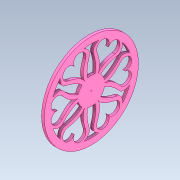
# Autodesk Inventor part: WheelFace
Saved by Autodesk Inventor 2021 (Build 250183000, 183)
## iProperties
Created: 2021-08-28
Part Number: WheelFace
Material: ABS Plastic
Document SubType Name: Modeling
Designer: digge
Density: 1.06 g/cm^3
Appearance: Pink
Author: digge
Autodesk Inventor part; units mm, degrees
ref_plane "YZ Plane" through (0, 0, 0) normal (1, 0, 0) x (0, 1, 0)
ref_plane "XZ Plane" through (0, 0, 0) normal (0, 1, 0) x (-1, 0, 0)
ref_plane "XY Plane" through (0, 0, 0) normal (0, 0, 1) x (1, 0, 0)
sketch "Sketch1" plane through (0, 0, 0) normal (1, 0, 0) x (0, 1, 0)
  circle A0 centre (168, 158) radius 175
  circle A1 centre (168, 158) radius 1.5
  point P0 (0, 0)
  dimension "d0" = 3
  dimension "d1" = 350
  constraints: 2 centre point, 1 coincident
  measures "d0" diameter of A1
  measures "d1" diameter of A0
extrude "Extrusion1" add sketch "Sketch1" along normal blind 10
sketch "Sketch2" plane through (10, 168, 158) normal (1, 0, 0) x (0, 0, -1)
  circle A0 centre (0, 0) radius 175 projected
  circle A1 centre (0, 0) radius 175 projected
  circle A2 centre (0, 0) radius 1.5 projected
  line L0 (-151.5544, 87.5) -> (0, 175) construction
  line L1 (0, 175) -> (151.5544, 87.5) construction
  line L2 (151.5544, 87.5) -> (151.5544, -87.5) construction
  line L3 (151.5544, -87.5) -> (0, -175) construction
  line L4 (0, -175) -> (-151.5544, -87.5) construction
  line L5 (-151.5544, -87.5) -> (-151.5544, 87.5) construction
  line L6 (0, -175) -> (0, 175) construction
  line L7 (-151.5544, -87.5) -> (151.5544, 87.5) construction
  line L8 (151.5544, -87.5) -> (-151.5544, 87.5) construction
  circle A3 centre (0, 0) radius 50 construction
  circle A4 centre (0, 0) radius 151.5544 construction
  line L9 (-151.5544, 0) -> (0, 0) construction
  line L10 (-54.4053, -31.4109) -> (-151.5544, -87.5) construction
  line L11 (-102.9799, -59.4555) -> (-102.9799, 59.4555) construction
  circle A5 centre (-126.2073, -23.2275) radius 23.2275 construction
  circle A6 centre (-126.2073, 23.2275) radius 23.2275 construction
  line L12 (-50, 0) -> (-75.7772, 0) construction
  line L13 (-75.7772, 0) -> (-108.5555, 38.3247) construction
  spline S0 degree 2 poles (-50, 0) (-75.7772, 0) (-108.5555, 38.3247) knots 1 1 1 2 2 2
  line L14 (-102.9799, 59.4555) -> (-102.9799, -59.4555) construction
  line L15 (-50, 0) -> (-75.7772, 0) construction
  line L16 (-75.7772, 0) -> (-108.5555, -38.3247) construction
  spline S1 degree 2 poles (-50, 0) (-75.7772, 0) (-108.5555, -38.3247) knots 1 1 1 2 2 2
  arc A7 (-126.2073, 0) -> (-108.5555, -38.3247) centre (-126.2073, -23.2275) ccw
  arc A8 (-108.5555, 38.3247) -> (-126.2073, 0) centre (-126.2073, 23.2275) ccw
  circle A9 centre (0, 0) radius 151.5544 construction
  circle A10 centre (-42.9881, 120.9125) radius 23.2275 construction
  circle A11 centre (-83.2193, 97.685) radius 23.2275 construction
  line L17 (-25, 43.3013) -> (-37.8886, 65.625) construction
  line L18 (-37.8886, 65.625) -> (-87.4679, 74.8494) construction
  spline S2 degree 2 poles (-25, 43.3013) (-37.8886, 65.625) (-87.4679, 74.8494) knots 1 1 1 2 2 2
  spline S3 degree 2 poles (-25, 43.3013) (-37.8886, 65.625) (-21.0875, 113.1741) knots 1 1 1 2 2 2
  line L19 (-37.8886, 65.625) -> (-21.0875, 113.1741) construction
  line L20 (-25, 43.3013) -> (-37.8886, 65.625) construction
  arc A12 (-21.0875, 113.1741) -> (-63.1037, 109.2988) centre (-42.9881, 120.9125) ccw
  arc A13 (-63.1037, 109.2988) -> (-87.4679, 74.8494) centre (-83.2193, 97.685) ccw
  line L21 (37.8886, 65.625) -> (21.0875, 113.1741) construction
  spline S4 degree 2 poles (25, 43.3013) (37.8886, 65.625) (21.0875, 113.1741) knots 1 1 1 2 2 2
  line L22 (25, 43.3013) -> (37.8886, 65.625) construction
  line L23 (37.8886, 65.625) -> (87.4679, 74.8494) construction
  spline S5 degree 2 poles (25, 43.3013) (37.8886, 65.625) (87.4679, 74.8494) knots 1 1 1 2 2 2
  line L24 (25, 43.3013) -> (37.8886, 65.625) construction
  circle A14 centre (83.2193, 97.685) radius 23.2275 construction
  arc A15 (87.4679, 74.8494) -> (63.1037, 109.2988) centre (83.2193, 97.685) ccw
  circle A16 centre (42.9881, 120.9125) radius 23.2275 construction
  arc A17 (63.1037, 109.2988) -> (21.0875, 113.1741) centre (42.9881, 120.9125) ccw
  line L25 (50, 0) -> (75.7772, 0) construction
  spline S6 degree 2 poles (50, 0) (75.7772, 0) (108.5555, -38.3247) knots 1 1 1 2 2 2
  line L26 (75.7772, 0) -> (108.5555, -38.3247) construction
  line L27 (50, 0) -> (75.7772, 0) construction
  spline S7 degree 2 poles (50, 0) (75.7772, 0) (108.5555, 38.3247) knots 1 1 1 2 2 2
  line L28 (75.7772, 0) -> (108.5555, 38.3247) construction
  circle A18 centre (126.2073, 23.2275) radius 23.2275 construction
  arc A19 (126.2073, 0) -> (108.5555, 38.3247) centre (126.2073, 23.2275) ccw
  circle A20 centre (126.2073, -23.2275) radius 23.2275 construction
  arc A21 (108.5555, -38.3247) -> (126.2073, 0) centre (126.2073, -23.2275) ccw
  line L29 (25, -43.3013) -> (37.8886, -65.625) construction
  spline S8 degree 2 poles (25, -43.3013) (37.8886, -65.625) (21.0875, -113.1741) knots 1 1 1 2 2 2
  line L30 (37.8886, -65.625) -> (21.0875, -113.1741) construction
  spline S9 degree 2 poles (25, -43.3013) (37.8886, -65.625) (87.4679, -74.8494) knots 1 1 1 2 2 2
  line L31 (25, -43.3013) -> (37.8886, -65.625) construction
  line L32 (37.8886, -65.625) -> (87.4679, -74.8494) construction
  circle A22 centre (83.2193, -97.685) radius 23.2275 construction
  arc A23 (63.1037, -109.2988) -> (87.4679, -74.8494) centre (83.2193, -97.685) ccw
  circle A24 centre (42.9881, -120.9125) radius 23.2275 construction
  arc A25 (21.0875, -113.1741) -> (63.1037, -109.2988) centre (42.9881, -120.9125) ccw
  line L33 (-25, -43.3013) -> (-37.8886, -65.625) construction
  spline S10 degree 2 poles (-25, -43.3013) (-37.8886, -65.625) (-21.0875, -113.1741) knots 1 1 1 2 2 2
  line L34 (-37.8886, -65.625) -> (-21.0875, -113.1741) construction
  line L35 (-25, -43.3013) -> (-37.8886, -65.625) construction
  spline S11 degree 2 poles (-25, -43.3013) (-37.8886, -65.625) (-87.4679, -74.8494) knots 1 1 1 2 2 2
  line L36 (-37.8886, -65.625) -> (-87.4679, -74.8494) construction
  circle A26 centre (-42.9881, -120.9125) radius 23.2275 construction
  arc A27 (-63.1037, -109.2988) -> (-21.0875, -113.1741) centre (-42.9881, -120.9125) ccw
  arc A28 (-87.4679, -74.8494) -> (-63.1037, -109.2988) centre (-83.2193, -97.685) ccw
  line L37 (0, 118.9109) -> (-102.9799, 59.4555) construction
  line L38 (0, 118.9109) -> (102.9799, 59.4555) construction
  line L39 (102.9799, -59.4555) -> (102.9799, 59.4555) construction
  line L40 (102.9799, -59.4555) -> (0, -118.9109) construction
  line L41 (-102.9799, -59.4555) -> (0, -118.9109) construction
  circle A29 centre (0, 0) radius 50 construction
  circle A30 centre (0, 0) radius 50 construction
  circle A31 centre (-83.2193, -97.685) radius 23.2275 construction
  circle A32 centre (0, 0) radius 50 construction
  circle A33 centre (0, 0) radius 50 construction
  circle A34 centre (0, 0) radius 50 construction
  circle A35 centre (0, 0) radius 50 construction
  circle A36 centre (0, 0) radius 50 construction
  circle A37 centre (0, 0) radius 50 construction
  circle A38 centre (0, 0) radius 50 construction
  circle A39 centre (0, 0) radius 50 construction
  circle A40 centre (0, 0) radius 50 construction
  circle A41 centre (0, 0) radius 50 construction
  circle A42 centre (0, 0) radius 50 construction
  circle A43 centre (0, 0) radius 50 construction
  circle A44 centre (0, 0) radius 50 construction
  circle A45 centre (0, 0) radius 50 construction
  circle A46 centre (0, 0) radius 151.5544 construction
  circle A47 centre (0, 0) radius 1.5 projected
  line L42 (-48.5263, -12.05) -> (-75.7772, -20) construction
  line L43 (-75.7772, -20) -> (-102.9799, -50) construction
  spline S12 degree 2 poles (-48.5263, -12.05) (-75.7772, -20) (-102.9799, -50) knots 1 1 1 2 2 2
  line L44 (-102.9799, -50) -> (-116.1046, -67.033) construction
  line L45 (-116.1046, -67.033) -> (-142.5144, -51.5596) construction
  spline S13 degree 2 poles (-102.9799, -50) (-116.1046, -67.033) (-142.5144, -51.5596) knots 1 1 1 2 2 2
  arc A48 (-142.5144, -51.5596) -> (-131.25, -75.7772) centre (0, 0) ccw
  circle A49 centre (0, 0) radius 151.5544 construction
  line L46 (-34.6987, -36) -> (-55.2091, -55.625) construction
  line L47 (-55.2091, -55.625) -> (-94.7912, -64.1832) construction
  spline S14 degree 2 poles (-34.6987, -36) (-55.2091, -55.625) (-94.7912, -64.1832) knots 1 1 1 2 2 2
  line L48 (-94.7912, -64.1832) -> (-116.1046, -67.033) construction
  line L49 (-116.1046, -67.033) -> (-115.9091, -97.6413) construction
  spline S15 degree 2 poles (-94.7912, -64.1832) (-116.1046, -67.033) (-115.9091, -97.6413) knots 1 1 1 2 2 2
  arc A50 (-131.25, -75.7772) -> (-115.9091, -97.6413) centre (0, 0) ccw
  arc A51 (-48.5263, -12.05) -> (-34.6987, -36) centre (0, 0) ccw
  circle A52 centre (0, 0) radius 151.5544 construction
  line L50 (-48.5263, 12.05) -> (-75.7772, 20) construction
  line L51 (-75.7772, 20) -> (-102.9799, 50) construction
  spline S16 degree 2 poles (-48.5263, 12.05) (-75.7772, 20) (-102.9799, 50) knots 1 1 1 2 2 2
  line L52 (-102.9799, 50) -> (-116.1046, 67.033) construction
  line L53 (-116.1046, 67.033) -> (-142.5144, 51.5596) construction
  spline S17 degree 2 poles (-102.9799, 50) (-116.1046, 67.033) (-142.5144, 51.5596) knots 1 1 1 2 2 2
  arc A53 (-131.25, 75.7772) -> (-142.5144, 51.5596) centre (0, 0) ccw
  circle A54 centre (0, 0) radius 151.5544 construction
  arc A55 (-115.9091, 97.6413) -> (-131.25, 75.7772) centre (0, 0) ccw
  spline S18 degree 2 poles (-94.7912, 64.1832) (-116.1046, 67.033) (-115.9091, 97.6413) knots 1 1 1 2 2 2
  line L54 (-94.7912, 64.1832) -> (-116.1046, 67.033) construction
  line L55 (-116.1046, 67.033) -> (-115.9091, 97.6413) construction
  spline S19 degree 2 poles (-34.6987, 36) (-55.2091, 55.625) (-94.7912, 64.1832) knots 1 1 1 2 2 2
  line L56 (-34.6987, 36) -> (-55.2091, 55.625) construction
  line L57 (-55.2091, 55.625) -> (-94.7912, 64.1832) construction
  arc A56 (-34.6987, 36) -> (-48.5263, 12.05) centre (0, 0) ccw
  circle A57 centre (0, 0) radius 151.5544 construction
  line L58 (75.7772, 131.25) -> (0, 0) construction
  circle A58 centre (0, 0) radius 151.5544 construction
  circle A59 centre (0, 0) radius 151.5544 construction
  circle A60 centre (0, 0) radius 151.5544 construction
  arc A61 (13.8276, 48.05) -> (-13.8276, 48.05) centre (0, 0) ccw
  spline S20 degree 2 poles (-13.8276, 48.05) (-20.5681, 75.625) (-8.1887, 114.1832) knots 1 1 1 2 2 2
  line L59 (-13.8276, 48.05) -> (-20.5681, 75.625) construction
  line L60 (-20.5681, 75.625) -> (-8.1887, 114.1832) construction
  spline S21 degree 2 poles (-8.1887, 114.1832) (0, 134.066) (-26.6053, 149.2009) knots 1 1 1 2 2 2
  line L61 (-8.1887, 114.1832) -> (0, 134.066) construction
  line L62 (0, 134.066) -> (-26.6053, 149.2009) construction
  circle A62 centre (0, 0) radius 151.5544 construction
  circle A63 centre (0, 0) radius 151.5544 construction
  arc A64 (0, 151.5544) -> (-26.6053, 149.2009) centre (0, 0) ccw
  arc A65 (26.6053, 149.2009) -> (0, 151.5544) centre (0, 0) ccw
  spline S22 degree 2 poles (8.1887, 114.1832) (0, 134.066) (26.6053, 149.2009) knots 1 1 1 2 2 2
  line L63 (8.1887, 114.1832) -> (0, 134.066) construction
  line L64 (0, 134.066) -> (26.6053, 149.2009) construction
  spline S23 degree 2 poles (13.8276, 48.05) (20.5681, 75.625) (8.1887, 114.1832) knots 1 1 1 2 2 2
  line L65 (13.8276, 48.05) -> (20.5681, 75.625) construction
  line L66 (20.5681, 75.625) -> (8.1887, 114.1832) construction
  arc A66 (48.5263, 12.05) -> (34.6987, 36) centre (0, 0) ccw
  spline S24 degree 2 poles (48.5263, 12.05) (75.7772, 20) (102.9799, 50) knots 1 1 1 2 2 2
  line L67 (48.5263, 12.05) -> (75.7772, 20) construction
  line L68 (75.7772, 20) -> (102.9799, 50) construction
  spline S25 degree 2 poles (102.9799, 50) (116.1046, 67.033) (142.5144, 51.5596) knots 1 1 1 2 2 2
  line L69 (102.9799, 50) -> (116.1046, 67.033) construction
  line L70 (116.1046, 67.033) -> (142.5144, 51.5596) construction
  arc A67 (131.25, 75.7772) -> (115.9091, 97.6413) centre (0, 0) ccw
  arc A68 (142.5144, 51.5596) -> (131.25, 75.7772) centre (0, 0) ccw
  spline S26 degree 2 poles (94.7912, 64.1832) (116.1046, 67.033) (115.9091, 97.6413) knots 1 1 1 2 2 2
  line L71 (94.7912, 64.1832) -> (116.1046, 67.033) construction
  line L72 (116.1046, 67.033) -> (115.9091, 97.6413) construction
  spline S27 degree 2 poles (34.6987, 36) (55.2091, 55.625) (94.7912, 64.1832) knots 1 1 1 2 2 2
  line L73 (34.6987, 36) -> (55.2091, 55.625) construction
  line L74 (55.2091, 55.625) -> (94.7912, 64.1832) construction
  circle A69 centre (0, 0) radius 151.5544 construction
  circle A70 centre (0, 0) radius 151.5544 construction
  circle A71 centre (0, 0) radius 151.5544 construction
  circle A72 centre (0, 0) radius 151.5544 construction
  circle A73 centre (0, 0) radius 151.5544 construction
  circle A74 centre (0, 0) radius 151.5544 construction
  arc A75 (34.6987, -36) -> (48.5263, -12.05) centre (0, 0) ccw
  spline S28 degree 2 poles (48.5263, -12.05) (75.7772, -20) (102.9799, -50) knots 1 1 1 2 2 2
  line L75 (48.5263, -12.05) -> (75.7772, -20) construction
  line L76 (75.7772, -20) -> (102.9799, -50) construction
  spline S29 degree 2 poles (34.6987, -36) (55.2091, -55.625) (94.7912, -64.1832) knots 1 1 1 2 2 2
  line L77 (34.6987, -36) -> (55.2091, -55.625) construction
  line L78 (55.2091, -55.625) -> (94.7912, -64.1832) construction
  spline S30 degree 2 poles (102.9799, -50) (116.1046, -67.033) (142.5144, -51.5596) knots 1 1 1 2 2 2
  line L79 (102.9799, -50) -> (116.1046, -67.033) construction
  line L80 (116.1046, -67.033) -> (142.5144, -51.5596) construction
  spline S31 degree 2 poles (94.7912, -64.1832) (116.1046, -67.033) (115.9091, -97.6413) knots 1 1 1 2 2 2
  line L81 (94.7912, -64.1832) -> (116.1046, -67.033) construction
  line L82 (116.1046, -67.033) -> (115.9091, -97.6413) construction
  arc A76 (131.25, -75.7772) -> (142.5144, -51.5596) centre (0, 0) ccw
  arc A77 (115.9091, -97.6413) -> (131.25, -75.7772) centre (0, 0) ccw
  circle A78 centre (0, 0) radius 151.5544 construction
  circle A79 centre (0, 0) radius 151.5544 construction
  arc A80 (-13.8276, -48.05) -> (13.8276, -48.05) centre (0, 0) ccw
  spline S32 degree 2 poles (13.8276, -48.05) (20.5681, -75.625) (8.1887, -114.1832) knots 1 1 1 2 2 2
  line L83 (13.8276, -48.05) -> (20.5681, -75.625) construction
  line L84 (20.5681, -75.625) -> (8.1887, -114.1832) construction
  spline S33 degree 2 poles (-13.8276, -48.05) (-20.5681, -75.625) (-8.1887, -114.1832) knots 1 1 1 2 2 2
  line L85 (-13.8276, -48.05) -> (-20.5681, -75.625) construction
  line L86 (-20.5681, -75.625) -> (-8.1887, -114.1832) construction
  spline S34 degree 2 poles (-8.1887, -114.1832) (0, -134.066) (-26.6053, -149.2009) knots 1 1 1 2 2 2
  line L87 (-8.1887, -114.1832) -> (0, -134.066) construction
  line L88 (0, -134.066) -> (-26.6053, -149.2009) construction
  spline S35 degree 2 poles (8.1887, -114.1832) (0, -134.066) (26.6053, -149.2009) knots 1 1 1 2 2 2
  line L89 (8.1887, -114.1832) -> (0, -134.066) construction
  line L90 (0, -134.066) -> (26.6053, -149.2009) construction
  arc A81 (-26.6053, -149.2009) -> (0, -151.5544) centre (0, 0) ccw
  arc A82 (0, -151.5544) -> (26.6053, -149.2009) centre (0, 0) ccw
  point P0 (158, -168)
  point P1 (-149.0512, -27.4317)
  point P2 (-75.7772, 131.25)
  point P3 (0, 62.8218)
  point P4 (-50.769, 142.798)
  point P5 (-11.2673, 111.8364)
  point P6 (-30.5568, 69.858)
  point P7 (-83.2193, 97.685)
  point P8 (-45.2204, 61.392)
  point P9 (83.2193, 97.685)
  point P10 (75.7772, 131.25)
  point P11 (-54.4053, 31.4109)
  point P12 (0, 62.8218)
  point P13 (-26.6053, -149.2009)
  point P14 (142.5144, -51.5596)
  point P15 (142.5144, 51.5596)
  point P16 (-26.6053, 149.2009)
  point P17 (-115.9091, 97.6413)
  point P18 (-115.9091, -97.6413)
  dimension "d4" = 100
  constraints: 121 symmetric about line, 78 point on circle, 71 centre point, 48 coincident, 38 end point, 8 line through centre, 5 vertical, 4 point on line, 4 tangent, 3 midpoint, 2 horizontal, 2 vertical alignment, 1 collinear, 1 horizontal alignment, 1 perpendicular, 207 other
extrude "Extrusion2" cut sketch "Sketch2" against normal through all contours S1 A7 A8 S0 | S2 A13 A12 S3 | S4 A17 A15 S5 | S7 A19 A21 S6 | S9 A23 A25 S8 | S10 A27 A28 S11 | A51 S14 S15 A50 A48 S13 S12 | S16 S17 A53 A55 S18 S19 A56 | A61 S20 S21 A64 A65 S22 S23 | A66 S27 S26 A67 A68 S25 S24 | A75 S28 S30 A76 A77 S31 S29 | A80 S32 S35 A82 A81 S34 S33
equation "\"d0\" = ScrewDiameter"
equation "\"d1\" = WheelDiameter"
equation "\"d2\" = Width"
equation "\"d4\" = CircleDiameter"
equation "\"WheelDiameter\" = 350"
equation "\"ScrewDiameter\" = 3"
equation "\"Width\" = 10"
equation "\"CircleDiameter\" = 100"
body "Solid1"
